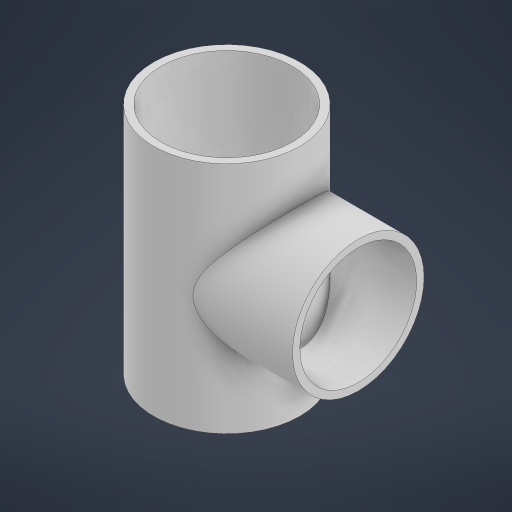
# Autodesk Inventor part: T Junction
Saved by Autodesk Inventor 2024.1 (Build 281209000, 209)
## iProperties
Created: 2024-11-18
Part Number: T Junction
Material: Generic
Document SubType Name: Modeling
Designer: Designer
Density: 1 g/cm^3
Appearance: Default
Author: Designer
Autodesk Inventor part; units mm, degrees
ref_plane "XZ Plane" through (0, 0, 0) normal (0, 1, 0) x (-1, 0, 0)
ref_plane "XY Plane" through (0, 0, 0) normal (0, 0, 1) x (1, 0, 0)
sketch "Sketch1" plane through (0, 0, 0) normal (0, 1, 0) x (-1, 0, 0)
  circle A0 centre (0, 0) radius 57.15
  circle A1 centre (0, 0) radius 63.5
  dimension "d0" = 114.3
  dimension "d1" = 6.35
  constraints: 2 centre point, 2 coincident
  measures "d0" diameter of A0
  measures "d1" radial gap between concentric circles of A0 A1
extrude "Extrusion1" add sketch "Sketch1" along normal blind 203.2
ref_plane "Work Plane1" through (63.5, 0, 0) normal (1, 0, 0) x (0, 1, 0)
sketch "Sketch2" plane through (63.5, 0, 0) normal (1, 0, 0) x (0, 1, 0)
  circle A0 centre (101.6, 0) radius 57.15
  circle A1 centre (101.6, 0) radius 50.8
  point P0 (0, 0)
  dimension "d4" = 101.6
  dimension "d5" = 114.3
  dimension "d6" = 101.6
  constraints: 2 centre point, 1 coincident
  measures "d4" distance of point (0, 0) A0.centre
  measures "d5" diameter of A0
  measures "d6" diameter of A1
extrude "Extrusion2" add sketch "Sketch2" along normal blind 50.8 and the other way blind 63.5
sketch "Sketch3" plane through (0, 203.2, 0) normal (0, 1, 0) x (1, 0, 0)
  circle A0 centre (0, 0) radius 57.15 projected
extrude "Extrusion3" cut sketch "Sketch3" against normal blind 254
body "Solid1"
